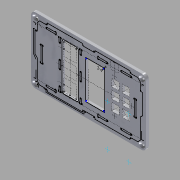
# Autodesk Inventor part: AK-C-C39-Top
Saved by Autodesk Inventor 2016 (Build 200138000, 138)
## iProperties
Created: 2016-04-01
Part Number: AK-C-C39-Top
Material: Aluminum 6061
Document SubType Name: Modeling
Designer: admin
Density: 2.7 g/cm^3
Appearance: Aluminum - Flat
Author: admin
Autodesk Inventor part; units mm, degrees
ref_plane "YZ Plane" through (0, 0, 0) normal (1, 0, 0) x (0, 1, 0)
ref_plane "XZ Plane" through (0, 0, 0) normal (0, 1, 0) x (-1, 0, 0)
ref_plane "XY Plane" through (0, 0, 0) normal (0, 0, 1) x (1, 0, 0)
derived "AK-C-C39-Main-Board.ipt"
sketch "Sketch1" plane through (0, 0, 0) normal (0, 1, 0) x (-1, 0, 0)
  line L0 (-55, -17.425) -> (-56.5, -17.425)
  line L1 (-56.5, -17.425) -> (-56.5, -16.775)
  line L2 (-58.5, -16.775) -> (-58.5, -17.425)
  line L3 (-58.5, -17.425) -> (-60, -17.425)
  line L4 (-60, -29.925) -> (-60, -17.425)
  line L5 (-60, -16.775) -> (-60, 29.925)
  line L6 (55, -17.425) -> (56.5, -17.425)
  line L7 (58.5, -17.425) -> (60, -17.425)
  line L8 (60, -29.925) -> (60, -17.425)
  line L9 (60, -16.775) -> (60, 29.925)
  arc A0 (-52.7, -29.3928) -> (-53.5536, -29.0392) centre (-53.2, -29.3928) ccw
  arc A1 (-54.6142, -27.9786) -> (-54.9678, -27.125) centre (-54.9678, -27.625) ccw
  line L10 (-54.0511, -29.5368) -> (-53.5536, -29.0392)
  line L11 (-55.1118, -28.4761) -> (-54.6142, -27.9786)
  arc A2 (54.6142, 27.9786) -> (54.9678, 27.125) centre (54.9678, 27.625) ccw
  line L12 (55.5, 29.925) -> (49.0175, 23.4425) construction
  arc A3 (52.7, 29.3928) -> (53.5536, 29.0392) centre (53.2, 29.3928) ccw
  line L13 (55, -16.775) -> (56.5, -16.775)
  line L14 (58.5, -16.775) -> (60, -16.775)
  line L15 (57.8, -3.3607) -> (55, -7.6074)
  line L16 (55, -7.6074) -> (55, -16.775)
  arc A4 (56.5, -18.525) -> (58.5, -18.525) centre (57.5, -19.275) ccw
  line L17 (58.5, -18.525) -> (58.5, -16.775)
  line L18 (56.5, -18.525) -> (56.5, -16.775)
  line L19 (-55.1118, 28.4761) -> (-54.6142, 27.9786)
  line L20 (-54.0059, 29.7916) -> (-53.5536, 29.3392)
  arc A5 (-53.5536, 29.3392) -> (-52.7, 29.6928) centre (-53.2, 29.6928) ccw
  arc A6 (-54.9678, 27.125) -> (-54.6142, 27.9786) centre (-54.9678, 27.625) ccw
  line L21 (-57.8, -3.3607) -> (-55, -7.6074)
  line L22 (-55, -7.6074) -> (-55, -16.775)
  arc A7 (-56.5, -15.025) -> (-58.5, -15.025) centre (-57.5, -14.275) ccw
  line L23 (-58.5, -15.025) -> (-58.5, -16.775)
  line L24 (-56.5, -15.025) -> (-56.5, -16.775)
  line L25 (-55, -16.775) -> (-56.5, -16.775)
  line L26 (-58.5, -16.775) -> (-60, -16.775)
  line L27 (57.5, -16.4962) -> (57.5, -11.7384) construction
  line L28 (-52.7, -31.925) -> (-52.7, -29.3928)
  line L29 (-54.9678, -27.125) -> (-57.5, -27.125)
  line L30 (-57.5, -27.125) -> (-57.5, -25.125)
  line L31 (-57.5, -25.125) -> (-55, -25.125)
  line L32 (-55, -25.125) -> (-55, -17.425)
  line L33 (48.7, -31.925) -> (46.7, -31.925)
  line L34 (46.7, -31.925) -> (46.7, -29.925)
  line L35 (46.7, -29.925) -> (44.7, -29.925)
  line L36 (44.7, -29.925) -> (44.7, -32.225)
  line L37 (-44.7, -32.225) -> (-44.7, -29.925)
  line L38 (-44.7, -29.925) -> (-46.7, -29.925)
  line L39 (-46.7, -29.925) -> (-46.7, -31.925)
  line L40 (-46.7, -31.925) -> (-48.7, -31.925)
  line L41 (-48.7, -31.925) -> (-48.7, -29.925)
  line L42 (-48.7, -29.925) -> (-50.7, -29.925)
  line L43 (-50.7, -29.925) -> (-50.7, -31.925)
  line L44 (-50.7, -31.925) -> (-52.7, -31.925)
  line L45 (55, -17.425) -> (55, -25.125)
  line L46 (55, -25.125) -> (57.5, -25.125)
  line L47 (57.5, -25.125) -> (57.5, -27.125)
  line L48 (57.5, -27.125) -> (54.9678, -27.125)
  line L49 (52.7, -29.3928) -> (52.7, -31.925)
  line L50 (52.7, -31.925) -> (50.7, -31.925)
  line L51 (50.7, -31.925) -> (50.7, -29.925)
  line L52 (50.7, -29.925) -> (48.7, -29.925)
  line L53 (48.7, -29.925) -> (48.7, -31.925)
  line L54 (5, -32.225) -> (5, -29.925)
  line L55 (5, -29.925) -> (3, -29.925)
  line L56 (3, -29.925) -> (3, -31.925)
  line L57 (3, -31.925) -> (1, -31.925)
  line L58 (1, -31.925) -> (1, -29.925)
  line L59 (1, -29.925) -> (-1, -29.925)
  line L60 (-1, -29.925) -> (-1, -31.925)
  line L61 (-1, -31.925) -> (-3, -31.925)
  line L62 (-3, -31.925) -> (-3, -29.925)
  line L63 (-3, -29.925) -> (-5, -29.925)
  line L64 (-5, -29.925) -> (-5, -32.225)
  line L65 (-5, -32.225) -> (-44.7, -32.225)
  line L66 (44.7, -32.225) -> (5, -32.225)
  line L67 (-57.5, -20.9142) -> (-57.5, -16.6435) construction
  arc A8 (60, 29.925) -> (55.5, 34.425) centre (55.5, 29.925) ccw
  arc A9 (-55.5, 34.425) -> (-60, 29.925) centre (-55.5, 29.925) ccw
  arc A10 (-60, -29.925) -> (-55.5, -34.425) centre (-55.5, -29.925) ccw
  line L68 (57.5, 27.125) -> (57.5, 25.125)
  line L69 (57.5, 25.125) -> (55.5, 25.125)
  line L70 (55.5, 25.125) -> (55.5, 23.125)
  line L71 (55.5, 23.125) -> (57.5, 23.125)
  line L72 (57.5, 23.125) -> (57.5, 21.125)
  line L73 (57.5, 21.125) -> (55.5, 21.125)
  line L74 (55.5, 21.125) -> (55.5, 19.125)
  line L75 (55.5, 19.125) -> (57.8, 19.125)
  line L76 (57.8, 19.125) -> (57.8, -3.3607)
  line L77 (3, 31.925) -> (1, 31.925)
  line L78 (1, 31.925) -> (1, 29.925)
  line L79 (1, 29.925) -> (-1, 29.925)
  line L80 (-1, 29.925) -> (-1, 31.925)
  line L81 (-1, 31.925) -> (-3, 31.925)
  line L82 (-3, 31.925) -> (-3, 29.925)
  line L83 (-3, 29.925) -> (-5, 29.925)
  line L84 (-5, 29.925) -> (-5, 32.225)
  line L85 (-5, 32.225) -> (-44.7, 32.225)
  line L86 (-44.7, 32.225) -> (-44.7, 29.925)
  line L87 (-44.7, 29.925) -> (-46.7, 29.925)
  line L88 (-46.7, 29.925) -> (-46.7, 32.225)
  line L89 (-46.7, 32.225) -> (-48.7, 32.225)
  line L90 (-48.7, 32.225) -> (-48.7, 29.925)
  line L91 (-48.7, 29.925) -> (-50.7, 29.925)
  line L92 (-50.7, 29.925) -> (-50.7, 32.225)
  line L93 (-50.7, 32.225) -> (-52.7, 32.225)
  line L94 (-52.7, 32.225) -> (-52.7, 29.6928)
  line L95 (-54.9678, 27.125) -> (-57.5, 27.125)
  line L96 (55.1118, 28.4761) -> (54.6142, 27.9786)
  line L97 (54.0511, 29.5368) -> (53.5536, 29.0392)
  line L98 (57.5, 27.125) -> (54.9678, 27.125)
  line L99 (52.7, 29.3928) -> (52.7, 31.925)
  line L100 (52.7, 31.925) -> (50.7, 31.925)
  line L101 (50.7, 31.925) -> (50.7, 29.925)
  line L102 (50.7, 29.925) -> (48.7, 29.925)
  line L103 (48.7, 29.925) -> (48.7, 31.925)
  line L104 (48.7, 31.925) -> (46.7, 31.925)
  line L105 (46.7, 31.925) -> (46.7, 29.925)
  line L106 (46.7, 29.925) -> (44.7, 29.925)
  line L107 (44.7, 29.925) -> (44.7, 32.225)
  line L108 (44.7, 32.225) -> (5, 32.225)
  line L109 (5, 32.225) -> (5, 29.925)
  line L110 (5, 29.925) -> (3, 29.925)
  line L111 (3, 29.925) -> (3, 31.925)
  line L112 (-57.5, 27.125) -> (-57.5, 25.125)
  line L113 (-57.5, 25.125) -> (-55.5, 25.125)
  line L114 (-55.5, 25.125) -> (-55.5, 23.125)
  line L115 (-55.5, 23.125) -> (-57.5, 23.125)
  line L116 (-57.5, 23.125) -> (-57.5, 21.125)
  line L117 (-57.5, 21.125) -> (-55.5, 21.125)
  line L118 (-55.5, 21.125) -> (-55.5, 19.125)
  line L119 (-55.5, 19.125) -> (-57.8, 19.125)
  line L120 (-57.8, 19.125) -> (-57.8, -3.3607)
  line L121 (55.5, -34.425) -> (-55.5, -34.425)
  line L122 (33.1179, 0) -> (-42.957, 0) construction
  line L123 (0, -20.0068) -> (0, 12.0803) construction
  line L124 (-77.7331, -29.925) -> (-117.8042, -29.925) construction
  line L125 (-91.6184, 29.925) -> (-122.9166, 29.925) construction
  line L126 (55.5, -18.8016) -> (55.5, 12.0803) construction
  line L127 (-55.5, -18.8016) -> (-55.5, 16.5996) construction
  arc A11 (55.5, -34.425) -> (60, -29.925) centre (55.5, -29.925) ccw
  arc A12 (54.9678, -27.125) -> (54.6142, -27.9786) centre (54.9678, -27.625) ccw
  arc A13 (53.5536, -29.0392) -> (52.7, -29.3928) centre (53.2, -29.3928) ccw
  line L128 (54.6142, -27.9786) -> (55.1118, -28.4761)
  line L129 (53.5536, -29.0392) -> (54.0511, -29.5368)
  arc A14 (55.1118, 28.4761) -> (54.0511, 29.5368) centre (55.5, 29.925) ccw
  arc A15 (-54.0059, 29.7916) -> (-55.1118, 28.4761) centre (-55.5, 29.925) ccw
  arc A16 (54.0511, -29.5368) -> (55.1118, -28.4761) centre (55.5, -29.925) ccw
  arc A17 (-55.1118, -28.4761) -> (-54.0511, -29.5368) centre (-55.5, -29.925) ccw
  line L130 (55.5, 34.425) -> (-55.5, 34.425)
  point P0 (0, 0)
sketch "Sketch2" plane through (0, 0, 0) normal (0, 1, 0) x (-1, 0, 0)
  line L0 (51.25, -29) -> (44, -29)
  line L1 (43.25, -29.75) -> (43.25, -31)
  line L2 (43.25, -31) -> (6.5, -31)
  line L3 (6.5, -31) -> (6.5, -29.75)
  line L4 (5.75, -29) -> (-5.75, -29)
  line L5 (-6.5, -29.75) -> (-6.5, -31)
  line L6 (-6.5, -31) -> (-43.25, -31)
  line L7 (-43.25, -31) -> (-43.25, -29.75)
  line L8 (-44, -29) -> (-51.25, -29)
  line L9 (-51.25, -29) -> (-53.75, -26.5)
  line L10 (-53.75, -26.5) -> (-53.75, -5.5)
  line L11 (-53.75, -5.5) -> (-56.25, -3)
  line L12 (-56.25, -3) -> (-56.25, 18)
  line L13 (-56.25, 18) -> (-54.5, 18)
  line L14 (-53.75, 18.75) -> (-53.75, 26.5)
  line L15 (-53.75, 26.5) -> (-51.25, 29)
  line L16 (-51.25, 29) -> (-44, 29)
  line L17 (-43.25, 29.75) -> (-43.25, 31)
  line L18 (-43.25, 31) -> (-6.5, 31)
  line L19 (-6.5, 31) -> (-6.5, 29.75)
  line L20 (-5.75, 29) -> (5.75, 29)
  line L21 (6.5, 29.75) -> (6.5, 31)
  line L22 (43.25, 31) -> (43.25, 29.75)
  line L23 (43.25, 31) -> (6.5, 31)
  line L24 (44, 29) -> (51.25, 29)
  line L25 (51.25, 29) -> (53.75, 26.5)
  line L26 (53.75, 26.5) -> (53.75, 18.75)
  line L27 (54.5, 18) -> (56.25, 18)
  line L28 (56.25, 18) -> (56.25, -3)
  line L29 (56.25, -3) -> (53.75, -5.5)
  line L30 (53.75, -5.5) -> (53.75, -26.5)
  line L31 (53.75, -26.5) -> (51.25, -29)
  line L32 (44.7, -32.225) -> (5, -32.225)
  line L33 (5, -32.225) -> (5, -29.925)
  line L34 (5, -29.925) -> (3, -29.925)
  line L35 (44.7, -29.925) -> (44.7, -32.225)
  line L36 (46.7, -29.925) -> (44.7, -29.925)
  line L37 (52.7, -29.3928) -> (52.7, -31.925)
  arc A0 (53.5536, -29.0392) -> (52.7, -29.3928) centre (53.2, -29.3928) ccw
  arc A1 (54.9678, -27.125) -> (54.6142, -27.9786) centre (54.9678, -27.625) ccw
  line L38 (55, -17.425) -> (55, -25.125)
  line L39 (0, -20.0068) -> (0, 12.0803) construction
  line L40 (33.1179, 0) -> (-42.957, 0) construction
  line L41 (57.8, 19.125) -> (57.8, -3.3607)
  line L42 (57.8, -3.3607) -> (55, -7.6074)
  line L43 (55.5, 19.125) -> (57.8, 19.125)
  line L44 (55.5, 29.925) -> (49.0175, 23.4425) construction
  line L45 (25.75, -24.5) -> (12.75, -24.5)
  line L46 (12.75, 24.5) -> (25.75, 24.5)
  line L47 (3.3524, -20) -> (-16.6476, -20)
  line L48 (-16.6476, -20) -> (-16.6476, 20)
  line L49 (-16.6476, 20) -> (3.3524, 20)
  line L50 (3.3524, 20) -> (3.3524, -20)
  line L51 (-23.9878, -15) -> (-31.9878, -15) construction
  line L52 (-31.9878, -15) -> (-31.9878, -7) construction
  line L53 (-31.9878, -7) -> (-23.9878, -7) construction
  line L54 (-23.9878, -7) -> (-23.9878, -15) construction
  line L55 (-34.9878, -15) -> (-42.9878, -15) construction
  line L56 (-42.9878, -15) -> (-42.9878, -7) construction
  line L57 (-42.9878, -7) -> (-34.9878, -7) construction
  line L58 (-34.9878, -7) -> (-34.9878, -15) construction
  line L59 (-23.9878, -4) -> (-31.9878, -4) construction
  line L60 (-31.9878, -4) -> (-31.9878, 4) construction
  line L61 (-31.9878, 4) -> (-23.9878, 4) construction
  line L62 (-23.9878, 4) -> (-23.9878, -4) construction
  line L63 (-34.9878, -4) -> (-42.9878, -4) construction
  line L64 (-42.9878, -4) -> (-42.9878, 4) construction
  line L65 (-42.9878, 4) -> (-34.9878, 4) construction
  line L66 (-34.9878, 4) -> (-34.9878, -4) construction
  line L67 (-23.9878, 7) -> (-31.9878, 7) construction
  line L68 (-31.9878, 7) -> (-31.9878, 15) construction
  line L69 (-31.9878, 15) -> (-23.9878, 15) construction
  line L70 (-23.9878, 15) -> (-23.9878, 7) construction
  line L71 (-34.9878, 7) -> (-42.9878, 7) construction
  line L72 (-42.9878, 7) -> (-42.9878, 15) construction
  line L73 (-42.9878, 15) -> (-34.9878, 15) construction
  line L74 (-34.9878, 15) -> (-34.9878, 7) construction
  line L75 (25.75, -22.5) -> (12.75, -22.5) construction
  line L76 (12.75, -22.5) -> (12.75, -9.5) construction
  line L77 (12.75, -9.5) -> (25.75, -9.5) construction
  line L78 (25.75, -9.5) -> (25.75, -22.5) construction
  line L79 (25.75, -6.5) -> (12.75, -6.5) construction
  line L80 (12.75, -6.5) -> (12.75, 6.5) construction
  line L81 (12.75, 6.5) -> (25.75, 6.5) construction
  line L82 (25.75, 6.5) -> (25.75, -6.5) construction
  line L83 (25.75, 9.5) -> (12.75, 9.5) construction
  line L84 (12.75, 9.5) -> (12.75, 22.5) construction
  line L85 (12.75, 22.5) -> (25.75, 22.5) construction
  line L86 (25.75, 22.5) -> (25.75, 9.5) construction
  line L87 (31.9633, -16) -> (17.7262, -16) construction
  line L88 (31.9633, 16) -> (18.8213, 16) construction
  line L89 (19.25, -23.7063) -> (19.25, 24.6931) construction
  arc A2 (10.75, -22.5) -> (12.75, -24.5) centre (12.75, -22.5) ccw
  arc A3 (25.75, -24.5) -> (27.75, -22.5) centre (25.75, -22.5) ccw
  arc A4 (12.75, 24.5) -> (10.75, 22.5) centre (12.75, 22.5) ccw
  arc A5 (27.75, 22.5) -> (25.75, 24.5) centre (25.75, 22.5) ccw
  line L90 (55, -25.125) -> (-54.9956, -25.125) construction
  line L91 (55.5, 25.125) -> (55.5, 23.125)
  line L92 (57.5, 25.125) -> (55.5, 25.125)
  line L93 (-57.5, 25.125) -> (-55.5, 25.125)
  line L94 (-55.5, 25.125) -> (-55.5, 23.125)
  line L95 (-57.5, -25.125) -> (-55, -25.125)
  line L96 (-55, -25.125) -> (-55, -17.425)
  line L97 (55, -25.125) -> (57.5, -25.125)
  line L98 (55.5, 25.125) -> (-55.5, 25.125) construction
  line L99 (48.25, -6.5) -> (48.25, 6.5)
  line L100 (50, -6.5) -> (50, 6.5)
  line L101 (50, -8) -> (48.25, -8)
  line L102 (50, 8) -> (48.25, 8)
  arc A6 (50, -8) -> (50, -6.5) centre (50, -7.25) ccw
  arc A7 (48.25, -6.5) -> (48.25, -8) centre (48.25, -7.25) ccw
  arc A8 (50, 6.5) -> (50, 8) centre (50, 7.25) ccw
  arc A9 (48.25, 8) -> (48.25, 6.5) centre (48.25, 7.25) ccw
  line L103 (-47.75, -6.5) -> (-47.75, 6.5)
  line L104 (-49.5, 8) -> (-47.75, 8)
  line L105 (-49.5, 6.5) -> (-49.5, -6.5)
  line L106 (-49.5, -8) -> (-47.75, -8)
  arc A10 (-47.75, -8) -> (-47.75, -6.5) centre (-47.75, -7.25) ccw
  arc A11 (-49.5, -6.5) -> (-49.5, -8) centre (-49.5, -7.25) ccw
  arc A12 (-47.75, 6.5) -> (-47.75, 8) centre (-47.75, 7.25) ccw
  arc A13 (-49.5, 8) -> (-49.5, 6.5) centre (-49.5, 7.25) ccw
  line L107 (43.75, -27) -> (35.5, -27)
  line L108 (33.75, -27) -> (33.75, -25.25)
  line L109 (35.5, -25.25) -> (43.75, -25.25)
  line L110 (-11, -27) -> (-19.25, -27)
  line L111 (-19.25, -25.25) -> (-11, -25.25)
  line L112 (-9.25, -25.25) -> (-9.25, -27)
  line L113 (-34.25, -27) -> (-44.25, -27)
  line L114 (-44.25, -25.25) -> (-34.25, -25.25)
  line L115 (-44.25, 25.25) -> (-34.25, 25.25)
  line L116 (-34.25, 27) -> (-44.25, 27)
  line L117 (-10.75, 25.25) -> (-19.25, 25.25)
  line L118 (-19.25, 27) -> (-10.75, 27)
  line L119 (-9.25, 27) -> (-9.25, 25.25)
  line L120 (43.75, 25.25) -> (35.25, 25.25)
  line L121 (33.75, 25.25) -> (33.75, 27)
  line L122 (35.25, 27) -> (43.75, 27)
  arc A14 (33.75, -27) -> (35.5, -27) centre (34.625, -27) ccw
  arc A15 (35.5, -25.25) -> (33.75, -25.25) centre (34.625, -25.25) ccw
  arc A16 (-11, -27) -> (-9.25, -27) centre (-10.125, -27) ccw
  arc A17 (-9.25, -25.25) -> (-11, -25.25) centre (-10.125, -25.25) ccw
  arc A18 (33.75, 25.25) -> (35.25, 25.25) centre (34.5, 25.25) ccw
  arc A19 (35.25, 27) -> (33.75, 27) centre (34.5, 27) ccw
  arc A20 (-9.25, 27) -> (-10.75, 27) centre (-10, 27) ccw
  arc A21 (-10.75, 25.25) -> (-9.25, 25.25) centre (-10, 25.25) ccw
  line L123 (27.75, 22.5) -> (27.75, -22.5)
  line L124 (-34.9878, 7) -> (-42.9878, 15) construction
  line L125 (-31.9878, 7) -> (-23.9878, 15) construction
  line L126 (-31.9878, -7) -> (-23.9878, -15) construction
  line L127 (-34.9878, -7) -> (-42.9878, -15) construction
  arc A22 (3.3524, 19) -> (2.3524, 20) centre (2.3524, 19) ccw
  arc A23 (-15.6476, 20) -> (-16.6476, 19) centre (-15.6476, 19) ccw
  arc A24 (2.3524, -20) -> (3.3524, -19) centre (2.3524, -19) ccw
  arc A25 (-16.6476, -19) -> (-15.6476, -20) centre (-15.6476, -19) ccw
  line L128 (10.75, 7.999) -> (10.75, 8)
  line L129 (10.75, -22.5) -> (10.75, 22.5)
  arc A26 (43.75, 25.25) -> (43.75, 27) centre (43.75, 26.125) ccw
  arc A27 (-19.25, 27) -> (-19.25, 25.25) centre (-19.25, 26.125) ccw
  arc A28 (-34.25, 25.25) -> (-34.25, 27) centre (-34.25, 26.125) ccw
  arc A29 (-44.25, 27) -> (-44.25, 25.25) centre (-44.25, 26.125) ccw
  arc A30 (43.75, -27) -> (43.75, -25.25) centre (43.75, -26.125) ccw
  arc A31 (-19.25, -25.25) -> (-19.25, -27) centre (-19.25, -26.125) ccw
  arc A32 (-34.25, -27) -> (-34.25, -25.25) centre (-34.25, -26.125) ccw
  arc A33 (-44.25, -25.25) -> (-44.25, -27) centre (-44.25, -26.125) ccw
  line L130 (31, 25) -> (29.25, 25)
  line L131 (31, 23.5) -> (31, 20)
  line L132 (29.25, 20) -> (29.25, 23.5)
  arc A34 (31, 23.5) -> (31, 25) centre (31, 24.25) ccw
  arc A35 (29.25, 25) -> (29.25, 23.5) centre (29.25, 24.25) ccw
  arc A36 (29.25, 20) -> (31, 20) centre (30.125, 20) ccw
  line L133 (29.25, -20) -> (29.25, -23.25)
  line L134 (29.25, -25) -> (31, -25)
  line L135 (31, -23.25) -> (31, -20)
  arc A37 (31, -25) -> (31, -23.25) centre (31, -24.125) ccw
  arc A38 (29.25, -23.25) -> (29.25, -25) centre (29.25, -24.125) ccw
  arc A39 (31, -20) -> (29.25, -20) centre (30.125, -20) ccw
  line L136 (9.25, 25) -> (7.5, 25)
  line L137 (7.5, 23.5) -> (7.5, 20)
  line L138 (9.25, 20) -> (9.25, 23.5)
  line L139 (7.5, -20) -> (7.5, -23.25)
  line L140 (7.5, -25) -> (9.25, -25)
  line L141 (9.25, -23.25) -> (9.25, -20)
  arc A40 (9.25, -20) -> (7.5, -20) centre (8.375, -20) ccw
  arc A41 (9.25, -25) -> (9.25, -23.25) centre (9.25, -24.125) ccw
  arc A42 (7.5, -23.25) -> (7.5, -25) centre (7.5, -24.125) ccw
  arc A43 (7.5, 20) -> (9.25, 20) centre (8.375, 20) ccw
  arc A44 (9.25, 23.5) -> (9.25, 25) centre (9.25, 24.25) ccw
  arc A45 (7.5, 25) -> (7.5, 23.5) centre (7.5, 24.25) ccw
  line L142 (29.25, 4) -> (29.25, -4)
  line L143 (31, -4) -> (31, 4)
  line L144 (7.5, 4) -> (7.5, -4)
  line L145 (9.25, -4) -> (9.25, 4)
  arc A46 (31, 4) -> (29.25, 4) centre (30.125, 4) ccw
  arc A47 (29.25, -4) -> (31, -4) centre (30.125, -4) ccw
  arc A48 (9.25, 4) -> (7.5, 4) centre (8.375, 4) ccw
  arc A49 (7.5, -4) -> (9.25, -4) centre (8.375, -4) ccw
  line L146 (-22.75, 30.3253) -> (-30.75, 30.3253) construction
  line L147 (-30.75, 30.3253) -> (-30.75, 22.4164) construction
  line L148 (-30.75, 22.4164) -> (-22.75, 22.4164) construction
  line L149 (-22.75, 22.4164) -> (-22.75, 30.3253) construction
  line L150 (-26.75, 29.9722) -> (-26.75, 20.9797) construction
  arc A50 (6.5, -29.75) -> (5.75, -29) centre (5.75, -29.75) ccw
  arc A51 (-5.75, -29) -> (-6.5, -29.75) centre (-5.75, -29.75) ccw
  arc A52 (-43.25, -29.75) -> (-44, -29) centre (-44, -29.75) ccw
  arc A53 (-54.5, 18) -> (-53.75, 18.75) centre (-54.5, 18.75) ccw
  arc A54 (-44, 29) -> (-43.25, 29.75) centre (-44, 29.75) ccw
  arc A55 (-6.5, 29.75) -> (-5.75, 29) centre (-5.75, 29.75) ccw
  arc A56 (5.75, 29) -> (6.5, 29.75) centre (5.75, 29.75) ccw
  arc A57 (43.25, 29.75) -> (44, 29) centre (44, 29.75) ccw
  arc A58 (53.75, 18.75) -> (54.5, 18) centre (54.5, 18.75) ccw
  arc A59 (44, -29) -> (43.25, -29.75) centre (44, -29.75) ccw
  line L151 (57.5, 27.125) -> (57.5, 25.125)
  line L152 (-57.5, 27.125) -> (-57.5, 25.125)
  point P0 (25.75, -16)
  point P1 (25.75, 16)
  point P2 (19.25, -22.5)
  point P3 (19.25, -24.5)
  point P4 (27.75, 0)
  point P5 (10.75, 0)
  point P6 (-26.75, 30.3253)
  point P7 (-26.75, 18)
  point P8 (-26.75, -18)
  point P9 (-44.75, 0)
  dimension "d33" = 2
  measures "d33" diameter of A23
sketch "Sketch3" plane through (0, 0, 0) normal (0, 1, 0) x (-1, 0, 0)
  line L0 (55.5, -34.425) -> (-55.5, -34.425) projected
  arc A0 (55.5, -34.425) -> (60, -29.925) centre (55.5, -29.925) ccw projected
  line L1 (60, -29.925) -> (60, -17.425) projected
  line L2 (60, -16.775) -> (60, 29.925) projected
  arc A1 (60, 29.925) -> (55.5, 34.425) centre (55.5, 29.925) ccw projected
  line L3 (55.5, 34.425) -> (-55.5, 34.425) projected
  arc A2 (-55.5, 34.425) -> (-60, 29.925) centre (-55.5, 29.925) ccw projected
  line L4 (-60, -16.775) -> (-60, 29.925) projected
  line L5 (-60, -29.925) -> (-60, -17.425) projected
  arc A3 (-60, -29.925) -> (-55.5, -34.425) centre (-55.5, -29.925) ccw projected
  line L6 (60, -17.425) -> (60, -16.775)
  line L7 (-60, -17.425) -> (-60, -16.775)
  point P0 (0, 0)
  constraints: 4 end point, 1 parallel, 1 vertical
extrude "Extrusion1" add sketch "Sketch3" along normal blind 3
hole "Hole1" at (-55.5, 0, 29.925) at (55.5, 0, 29.925) at (-55.5, 0, -29.925) at (55.5, 0, -29.925) direction (0, 1, 0) diameter 3 end through all countersink diameter 6 countersink angle 90
extrude "Extrusion3" cut sketch "Sketch2" along normal blind 3 contours L47 A25 L48 A23 L49 A22 L50 A24
sketch "Sketch5" plane through (0, 0, 0) normal (0, -1, 0) x (1, 0, 0)
  line L0 (23.9878, 15) -> (23.9878, 7) projected
  line L1 (31.9878, 15) -> (23.9878, 15) projected
  line L2 (31.9878, 7) -> (31.9878, 15) projected
  line L3 (23.9878, 7) -> (31.9878, 7) projected
  line L4 (31.9878, 4) -> (23.9878, 4) projected
  line L5 (23.9878, 4) -> (23.9878, -4) projected
  line L6 (23.9878, -4) -> (31.9878, -4) projected
  line L7 (31.9878, -4) -> (31.9878, 4) projected
  line L8 (31.9878, -7) -> (23.9878, -7) projected
  line L9 (23.9878, -7) -> (23.9878, -15) projected
  line L10 (23.9878, -15) -> (31.9878, -15) projected
  line L11 (31.9878, -15) -> (31.9878, -7) projected
  line L12 (34.9878, -7) -> (34.9878, -15) projected
  line L13 (34.9878, -15) -> (42.9878, -15) projected
  line L14 (42.9878, -15) -> (42.9878, -7) projected
  line L15 (42.9878, -7) -> (34.9878, -7) projected
  line L16 (34.9878, -4) -> (42.9878, -4) projected
  line L17 (34.9878, 4) -> (34.9878, -4) projected
  line L18 (42.9878, 4) -> (34.9878, 4) projected
  line L19 (42.9878, -4) -> (42.9878, 4) projected
  line L20 (42.9878, 7) -> (42.9878, 15) projected
  line L21 (42.9878, 15) -> (34.9878, 15) projected
  line L22 (34.9878, 15) -> (34.9878, 7) projected
  line L23 (34.9878, 7) -> (42.9878, 7) projected
  arc A0 (23.9878, -14) -> (24.9878, -15) centre (24.9878, -14) ccw
  arc A1 (24.9878, -7) -> (23.9878, -8) centre (24.9878, -8) ccw
  arc A2 (30.9878, -15) -> (31.9878, -14) centre (30.9878, -14) ccw
  arc A3 (31.9878, -8) -> (30.9878, -7) centre (30.9878, -8) ccw
  arc A4 (34.9878, -14) -> (35.9878, -15) centre (35.9878, -14) ccw
  arc A5 (35.9878, -7) -> (34.9878, -8) centre (35.9878, -8) ccw
  arc A6 (41.9878, -15) -> (42.9878, -14) centre (41.9878, -14) ccw
  arc A7 (42.9878, -8) -> (41.9878, -7) centre (41.9878, -8) ccw
  arc A8 (34.9878, -3) -> (35.9878, -4) centre (35.9878, -3) ccw
  arc A9 (35.9878, 4) -> (34.9878, 3) centre (35.9878, 3) ccw
  arc A10 (41.9878, -4) -> (42.9878, -3) centre (41.9878, -3) ccw
  arc A11 (42.9878, 3) -> (41.9878, 4) centre (41.9878, 3) ccw
  arc A12 (23.9878, -3) -> (24.9878, -4) centre (24.9878, -3) ccw
  arc A13 (24.9878, 4) -> (23.9878, 3) centre (24.9878, 3) ccw
  arc A14 (30.9878, -4) -> (31.9878, -3) centre (30.9878, -3) ccw
  arc A15 (31.9878, 3) -> (30.9878, 4) centre (30.9878, 3) ccw
  arc A16 (23.9878, 8) -> (24.9878, 7) centre (24.9878, 8) ccw
  arc A17 (24.9878, 15) -> (23.9878, 14) centre (24.9878, 14) ccw
  arc A18 (30.9878, 7) -> (31.9878, 8) centre (30.9878, 8) ccw
  arc A19 (31.9878, 14) -> (30.9878, 15) centre (30.9878, 14) ccw
  arc A20 (34.9878, 8) -> (35.9878, 7) centre (35.9878, 8) ccw
  arc A21 (35.9878, 15) -> (34.9878, 14) centre (35.9878, 14) ccw
  arc A22 (41.9878, 7) -> (42.9878, 8) centre (41.9878, 8) ccw
  arc A23 (42.9878, 14) -> (41.9878, 15) centre (41.9878, 14) ccw
  point P0 (0, 0)
  dimension "d16" = 2
  constraints: 48 point on circle, 48 point on line, 48 tangent, 24 centre point, 23 equal radius
  measures "d16" diameter of A0
extrude "Extrusion5" cut sketch "Sketch5" against normal up to next contours A17 L1 A19 L2 A18 L3 A16 L0 | A15 L7 A14 L6 A12 L5 A13 L4 | A3 L11 A2 L10 A0 L9 A1 L8 | A5 L15 A7 L14 A6 L13 A4 L12 | A8 L17 A9 L18 A11 L19 A10 L16 | A22 L23 A20 L22 A21 L21 A23 L20
sketch "Sketch6" plane through (0, 0, 0) normal (0, -1, 0) x (1, 0, 0)
  point P0 (0, 0)
  point P1 (19.46, -8.4923)
  point P2 (26.75, 18)
  point P3 (44.75, 0)
  point P4 (26.75, -18)
hole "Hole3" at (26.75, 0, 18) at (44.75, 0, 0) at (26.75, 0, -18) direction (0, 1, 0) diameter 1.567 depth 35.169 tip angle 118 thread size "M2x0.4" class "6H" standard "ANSI Metric M Profile"
extrude "Extrusion6" cut sketch "Sketch2" along normal blind 10 contours L45 A2 L129 A4 L46 A5 L123 A3
body "Solid1"
